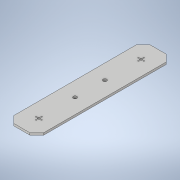
# Autodesk Inventor part: testPart_chassis2
Saved by Autodesk Inventor 2020 (Build 240168000, 168)
## iProperties
Created: 2019-09-17
Part Number: testPart_chassis2
Material: Generic
Document SubType Name: Modeling
Designer: shrey
Density: 1 g/cm^3
Appearance: Default
Author: shrey
Autodesk Inventor part; units mm, degrees
ref_plane "YZ Plane" through (0, 0, 0) normal (1, 0, 0) x (0, 1, 0)
ref_plane "XZ Plane" through (0, 0, 0) normal (0, 1, 0) x (-1, 0, 0)
ref_plane "XY Plane" through (0, 0, 0) normal (0, 0, 1) x (1, 0, 0)
sketch "Sketch1" plane through (0, 0, 0) normal (0, 1, 0) x (-1, 0, 0)
  line L0 (-44.45, -203.2) -> (44.45, -203.2)
  line L1 (44.45, -203.2) -> (44.45, 203.2)
  line L2 (44.45, 203.2) -> (-44.45, 203.2)
  line L3 (-44.45, 203.2) -> (-44.45, -203.2)
  line L4 (-44.45, -203.2) -> (44.45, 203.2) construction
  line L5 (44.45, -203.2) -> (-44.45, 203.2) construction
  line L6 (0, 203.2) -> (0, -203.2) construction
  line L7 (0, 0) -> (44.45, 0) construction
  line L8 (0, -203.2) -> (0, 203.2) construction
  line L9 (0, 152.4) -> (7.112, 152.4) construction
  line L10 (0, -152.4) -> (0, -203.2) construction
  circle A0 centre (0, -152.4) radius 4
  circle A1 centre (0, -152.4) radius 8 construction
  line L11 (0, 152.4) -> (-44.45, 152.4) construction
  line L12 (-44.45, 152.4) -> (-44.45, 88.9)
  line L13 (-44.45, 88.9) -> (0, 88.9) construction
  line L14 (0, 88.9) -> (0, 152.4) construction
  circle A2 centre (0, -144.4) radius 1.85
  circle A3 centre (-8, -152.4) radius 1.85
  circle A4 centre (0, -160.4) radius 1.85
  circle A5 centre (8, -152.4) radius 1.85
  circle A6 centre (0, 152.4) radius 4
  circle A7 centre (0, 152.4) radius 8 construction
  circle A8 centre (0, 160.4) radius 1.85
  circle A9 centre (0, 152.4) radius 8 construction
  circle A10 centre (-8, 152.4) radius 1.85
  circle A11 centre (0, 152.4) radius 8 construction
  circle A12 centre (0, 144.4) radius 1.85
  circle A13 centre (0, 152.4) radius 8 construction
  circle A14 centre (8, 152.4) radius 1.85
  line L15 (-88.9, 44.45) -> (0, 44.45) construction
  line L16 (0, 44.45) -> (0, -44.45) construction
  line L17 (0, -44.45) -> (-88.9, -44.45) construction
  line L18 (-88.9, -44.45) -> (-88.9, 44.45) construction
  line L19 (-88.9, 44.45) -> (0, -44.45) construction
  line L20 (0, 44.45) -> (-88.9, -44.45) construction
  circle A15 centre (0, 44.45) radius 5.5563
  circle A16 centre (0, -44.45) radius 5.5563
  point P0 (-44.45, 0)
  dimension "d17" = 16
  dimension "d40" = 16
  dimension "d0" = 406.4
  dimension "d1" = 88.9
  dimension "d2" = 152.4
  dimension "d16" = 8
  dimension "d24" = 44.45
  dimension "d25" = 63.5
  dimension "d34" = 3.7
  dimension "d37" = 360
  dimension "d39" = 8
  dimension "d41" = 3.7
  dimension "d44" = 360
  dimension "d63" = 88.9
  dimension "d64" = 11.1125
  dimension "d65" = 11.1125
  constraints: 42 end point, 12 centre point, 9 coincident, 8 midpoint, 6 parallel, 4 horizontal, 4 point on line, 3 perpendicular, 3 symmetric about line, 3 vertical alignment, 2 horizontal alignment, 1 collinear, 34 other
  measures "d0" distance of L0.end L1.end
  measures "d1" distance of L1.end L2.end
  measures "d2" distance of L7.start point (0, 152.4)
  measures "d16" diameter of A0
  measures "d24" distance of L9.start L11.end
  measures "d25" distance of L11.end L12.end
  measures "d34" diameter of A2
  measures "d39" diameter of A6
  measures "d41" diameter of A8
  measures "d63" distance of L17.end L15.start
  measures "d64" diameter of A15
  measures "d65" diameter of A16
extrude "Extrusion6" add sketch "Sketch1" along normal blind 6.35
chamfer "Chamfer6" distance 20.32 angle 45 4 edges at (-44.45, 3.175, 203.2) (44.45, 3.175, 203.2) (44.45, 3.175, -203.2) (-44.45, 3.175, -203.2)
body "Solid6"
